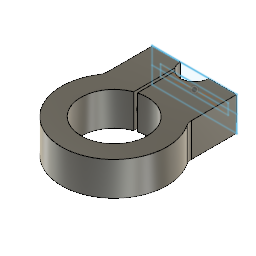
bmp280_bracket_OSft120 (Autodesk Fusion 360 design; units mm, degrees)
Autodesk Fusion 360 part; units mm, degrees
note: some values were not read from the file. Set by a fixed rule: which sketch regions a step uses.
sketch "Sketch1" plane through (0, 0, 0) normal (0, 0, 1) x (1, 0, 0)
  line L0 (-7.5, 14.2587) -> (-2.5, 14.2587)
  line L1 (-2.0653, 12.85) -> (-2.0653, 5.5267)
  arc A0 (-7.8282, 5.1403) -> (7.8282, 5.1403) centre (0, 0) ccw
  line L2 (-1.565, 12.3091) -> (-1.565, 5.6887)
  line L3 (-2.0653, 5.5267) -> (-2.0653, 12.85)
  line L4 (-7.5, 14.2587) -> (-2.5, 14.2587)
  line L5 (2.5, 14.2587) -> (7.5, 14.2587)
  arc A1 (-2.0653, 5.5267) -> (-1.565, 5.6887) centre (0, 0) ccw
  line L6 (-2.5, -19.9263) -> (2.5, -19.9263)
  arc A2 (-1.565, 12.3091) -> (2.5, 14.2587) centre (0, 14.2587) ccw
  arc A3 (-2.5, 14.2587) -> (-2.0653, 12.85) centre (0, 14.2587) ccw
  line L7 (0, 0) -> (-7.5, 0)
  line L8 (-7.5, 6.238) -> (-7.5, 14.2587)
  line L9 (0, 0) -> (7.5, 0)
  line L10 (7.5, 6.238) -> (7.5, 14.2587)
  line L11 (0, 17.4341) -> (0, 17.3504)
  arc A4 (-7.8282, 5.1403) -> (-7.5, 6.238) centre (-9.5, 6.238) ccw
  arc A5 (7.5, 6.238) -> (7.8282, 5.1403) centre (9.5, 6.238) ccw
  dimension "d1" = 11.8
  dimension "d5" = 5
  dimension "d25" = 7.5
  dimension "d26" = 7.5
  dimension "d27" = 2
  constraint coincident A0.centre A1.centre
  constraint horizontal L0
  constraint vertical L1
  constraint concentric A0 A1
  constraint vertical L2
  constraint vertical L3
  constraint collinear L4 L5
  constraint coincident L0.end A2
  constraint concentric A2 A3
  constraint horizontal L7
  constraint vertical L8
  constraint vertical L11
  constraint horizontal L9
  constraint vertical L10
  constraint tangent L8 A4
  constraint tangent A0 A4
  constraint tangent A0 A5
  constraint tangent L10 A5
  constraint equal A4 A5
  measures "d1" diameter of A1
  measures "d5" distance of L6.start L6.end
  measures "d25" distance of A0.centre L7.end
  measures "d26" distance of A0.centre L9.end
  measures "d27" radius of A4
extrude "Extrude1" add sketch "Sketch1" along normal blind 6 contours L0 L1 A0 L2 L3 L4 L5 A1 A2 A3 L8 L10 A4 A5
hole "Hole1" at (-7.5, 7.2587, 3) direction (1, 0, 0) diameter 2.4 depth 5.6892 tip angle 180
hole "Hole2" at (-1.565, 7.2768, 3) direction (1, 0, 0) diameter 1.5 depth 8.4147 tip angle 180
sketch "Sketch2" plane through (0, 14.2587, 0) normal (0, 1, 0) x (-1, 0, 0)
  line L0 (7.5233, 0) -> (-7.4993, 0)
  line L1 (-7.4993, 0) -> (-7.4993, 6.0044)
  line L2 (-7.4993, 6.0044) -> (7.5233, 6.0044)
  line L3 (7.5233, 6.0044) -> (7.5233, 0)
  line L4 (7.5233, 3.0022) -> (-7.4993, 3.0022)
  line L5 (6.012, 2.0757) -> (-5.988, 2.0757)
  line L6 (-5.988, 2.0757) -> (-5.988, 3.9288)
  line L7 (-5.988, 3.9288) -> (6.012, 3.9288)
  line L8 (6.012, 3.9288) -> (6.012, 2.0757)
  line L9 (6.012, 2.0757) -> (-5.988, 3.9288) construction
  line L10 (-5.988, 2.0757) -> (6.012, 3.9288) construction
  point P0 (0.012, 3.0022)
  dimension "d30" = 12
  constraint horizontal L0
  constraint vertical L1
  constraint horizontal L2
  constraint vertical L3
  constraint midpoint L3 L4.start
  constraint midpoint L1 L4.end
  constraint horizontal L5
  constraint perpendicular L5 L6
  constraint parallel L5 L7
  constraint parallel L6 L8
  constraint coincident L9 P0
  constraint coincident L10 P0
  constraint midpoint L4 P0
  measures "d30" distance of L6.end L7.end
hole "Hole3" at (5.991, 14.2587, 3.0012) direction (0, -1, 0) diameter 1.5 depth 5 tip angle 180
hole "Hole4" at (-6.0143, 14.2587, 3.0029) direction (0, -1, 0) diameter 1.5 depth 5 tip angle 180
